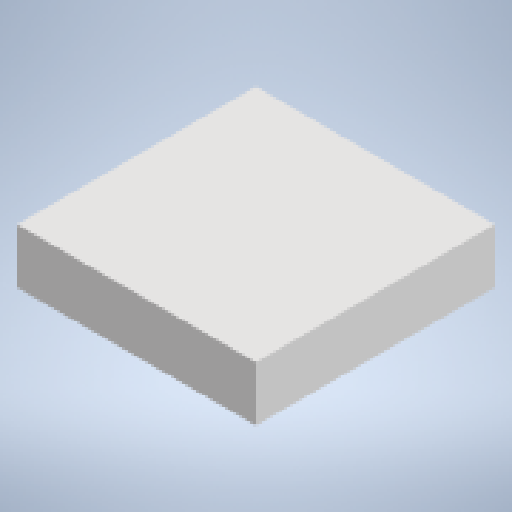
# Autodesk Inventor part: STOCK_MATERIAL_1
Saved by Autodesk Inventor 2023.2 (Build 272271030, 271C)
## iProperties
Created: 2023-08-30
Part Number: STOCK_MATERIAL_1
Material: Generic
Document SubType Name: Modeling
Designer: Cris Pat
Density: 1 g/cm^3
Appearance: Default
Author: Cris Pat
Autodesk Inventor part; units mm, degrees
ref_plane "YZ Plane" through (0, 0, 0) normal (1, 0, 0) x (0, 1, 0)
ref_plane "XZ Plane" through (0, 0, 0) normal (0, 1, 0) x (-1, 0, 0)
sketch "Sketch1" plane through (0, 0, 0) normal (0, 0, 1) x (1, 0, 0)
  line L0 (0, 0) -> (0, 76.2) construction
  line L1 (0, 76.2) -> (76.2, 76.2) construction
  line L2 (76.2, 76.2) -> (76.2, 0) construction
  line L3 (76.2, 0) -> (0, 0) construction
  line L4 (73.2, 73.2) -> (3, 73.2)
  line L5 (3, 73.2) -> (3, 3)
  line L6 (3, 3) -> (73.2, 3)
  line L7 (73.2, 3) -> (73.2, 73.2)
  dimension "d0" = 3
  constraints: 8 end point, 3 other
  measures "d0" distance between parallel lines of L1 L4
ref_plane "Work Plane1" through (-3.81, -3.81, -16.05) normal (0, 0, 1) x (1, 0, 0)
extrude "Extrusion1" add sketch "Sketch1" against normal up to surface (16.05 mm away)
body "Solid1"
